Autodesk Inventor part; units mm, degrees
(part 2 of 3)
  line L955 (15.8047, 2.9296) -> (15.8214, 3.0524)
  line L956 (15.8214, 3.0524) -> (15.8318, 3.1132)
  line L957 (15.8318, 3.1132) -> (15.8442, 3.1734)
  line L958 (15.8442, 3.1734) -> (15.5913, 3.315)
  line L959 (15.5913, 3.315) -> (15.2554, 3.4241)
  line L960 (15.2554, 3.4241) -> (14.9676, 3.4583)
  line L961 (14.9676, 3.4583) -> (14.9422, 3.4023)
  line L962 (14.9422, 3.4023) -> (14.915, 3.3469)
  line L963 (14.915, 3.3469) -> (14.8562, 3.2378)
  line L964 (14.8562, 3.2378) -> (14.7929, 3.1303)
  line L965 (14.7929, 3.1303) -> (14.7259, 3.0241)
  line L966 (14.7259, 3.0241) -> (14.5818, 2.8156)
  line L967 (14.5818, 2.8156) -> (14.4261, 2.6115)
  line L968 (14.4261, 2.6115) -> (14.2601, 2.4115)
  line L969 (14.2601, 2.4115) -> (14.0847, 2.2154)
  line L970 (14.0847, 2.2154) -> (13.9004, 2.0233)
  line L971 (13.9004, 2.0233) -> (13.7077, 1.8349)
  line L972 (13.7077, 1.8349) -> (13.507, 1.6503)
  line L973 (13.507, 1.6503) -> (13.3514, 1.5144)
  line L974 (13.3514, 1.5144) -> (12.8549, 1.72)
  line L975 (12.8549, 1.72) -> (12.841, 1.9262)
  line L976 (12.841, 1.9262) -> (12.8296, 2.1986)
  line L977 (12.8296, 2.1986) -> (12.8265, 2.4681)
  line L978 (12.8265, 2.4681) -> (12.8321, 2.7343)
  line L979 (12.8321, 2.7343) -> (12.8466, 2.997)
  line L980 (12.8466, 2.997) -> (12.8707, 3.2557)
  line L981 (12.8707, 3.2557) -> (12.9049, 3.5101)
  line L982 (12.9049, 3.5101) -> (12.9505, 3.7595)
  line L983 (12.9505, 3.7595) -> (12.9781, 3.882)
  line L984 (12.9781, 3.882) -> (13.0095, 4.0027)
  line L985 (13.0095, 4.0027) -> (13.0451, 4.1215)
  line L986 (13.0451, 4.1215) -> (13.0649, 4.1799)
  line L987 (13.0649, 4.1799) -> (13.0865, 4.2374)
  line L988 (13.0865, 4.2374) -> (12.8589, 4.4167)
  line L989 (12.8589, 4.4167) -> (12.5442, 4.5771)
  line L990 (12.5442, 4.5771) -> (12.2654, 4.6558)
  line L991 (12.2654, 4.6558) -> (12.2315, 4.6045)
  line L992 (12.2315, 4.6045) -> (12.1959, 4.5541)
  line L993 (12.1959, 4.5541) -> (12.1208, 4.4555)
  line L994 (12.1208, 4.4555) -> (12.0415, 4.3592)
  line L995 (12.0415, 4.3592) -> (11.9586, 4.2649)
  line L996 (11.9586, 4.2649) -> (11.7837, 4.0814)
  line L997 (11.7837, 4.0814) -> (11.5981, 3.9042)
  line L998 (11.5981, 3.9042) -> (11.4028, 3.7326)
  line L999 (11.4028, 3.7326) -> (11.1989, 3.5664)
  line L1000 (11.1989, 3.5664) -> (10.9868, 3.4055)
  line L1001 (10.9868, 3.4055) -> (10.7669, 3.2496)
  line L1002 (10.7669, 3.2496) -> (10.5398, 3.0987)
  line L1003 (10.5398, 3.0987) -> (10.3649, 2.9888)
  line L1004 (10.3649, 2.9888) -> (9.9067, 3.2695)
  line L1005 (9.9067, 3.2695) -> (9.9252, 3.4753)
  line L1006 (9.9252, 3.4753) -> (9.9566, 3.7462)
  line L1007 (9.9566, 3.7462) -> (9.9957, 4.0128)
  line L1008 (9.9957, 4.0128) -> (10.0428, 4.2749)
  line L1009 (10.0428, 4.2749) -> (10.0983, 4.532)
  line L1010 (10.0983, 4.532) -> (10.1625, 4.7839)
  line L1011 (10.1625, 4.7839) -> (10.2362, 5.0298)
  line L1012 (10.2362, 5.0298) -> (10.3202, 5.2689)
  line L1013 (10.3202, 5.2689) -> (10.3666, 5.3856)
  line L1014 (10.3666, 5.3856) -> (10.4164, 5.5)
  line L1015 (10.4164, 5.5) -> (10.4702, 5.6116)
  line L1016 (10.4702, 5.6116) -> (10.499, 5.6662)
  line L1017 (10.499, 5.6662) -> (10.5293, 5.7197)
  line L1018 (10.5293, 5.7197) -> (10.3326, 5.9324)
  line L1019 (10.3326, 5.9324) -> (10.0468, 6.14)
  line L1020 (10.0468, 6.14) -> (9.7837, 6.2614)
  line L1021 (9.7837, 6.2614) -> (9.7422, 6.216)
  line L1022 (9.7422, 6.216) -> (9.6992, 6.1718)
  line L1023 (9.6992, 6.1718) -> (9.6096, 6.0862)
  line L1024 (9.6096, 6.0862) -> (9.5162, 6.0035)
  line L1025 (9.5162, 6.0035) -> (9.4196, 5.9233)
  line L1026 (9.4196, 5.9233) -> (9.2181, 5.7694)
  line L1027 (9.2181, 5.7694) -> (9.007, 5.6234)
  line L1028 (9.007, 5.6234) -> (8.7874, 5.4845)
  line L1029 (8.7874, 5.4845) -> (8.5599, 5.3523)
  line L1030 (8.5599, 5.3523) -> (8.3252, 5.2265)
  line L1031 (8.3252, 5.2265) -> (8.0837, 5.1069)
  line L1032 (8.0837, 5.1069) -> (7.8358, 4.9934)
  line L1033 (7.8358, 4.9934) -> (7.6459, 4.9122)
  line L1034 (7.6459, 4.9122) -> (7.2372, 5.2611)
  line L1035 (7.2372, 5.2611) -> (7.2877, 5.4615)
  line L1036 (7.2877, 5.4615) -> (7.361, 5.7241)
  line L1037 (7.361, 5.7241) -> (7.4414, 5.9813)
  line L1038 (7.4414, 5.9813) -> (7.5289, 6.2328)
  line L1039 (7.5289, 6.2328) -> (7.6239, 6.4781)
  line L1040 (7.6239, 6.4781) -> (7.7268, 6.7168)
  line L1041 (7.7268, 6.7168) -> (7.838, 6.9482)
  line L1042 (7.838, 6.9482) -> (7.9584, 7.1712)
  line L1043 (7.9584, 7.1712) -> (8.0225, 7.2792)
  line L1044 (8.0225, 7.2792) -> (8.0896, 7.3844)
  line L1045 (8.0896, 7.3844) -> (8.1602, 7.4863)
  line L1046 (8.1602, 7.4863) -> (8.1971, 7.5357)
  line L1047 (8.1971, 7.5357) -> (8.2354, 7.5837)
  line L1048 (8.2354, 7.5837) -> (8.0744, 7.8246)
  line L1049 (8.0744, 7.8246) -> (7.8246, 8.0744)
  line L1050 (7.8246, 8.0744) -> (7.5837, 8.2354)
  line L1051 (7.5837, 8.2354) -> (7.5357, 8.1971)
  line L1052 (7.5357, 8.1971) -> (7.4863, 8.1602)
  line L1053 (7.4863, 8.1602) -> (7.3844, 8.0896)
  line L1054 (7.3844, 8.0896) -> (7.2792, 8.0225)
  line L1055 (7.2792, 8.0225) -> (7.1712, 7.9584)
  line L1056 (7.1712, 7.9584) -> (6.9482, 7.838)
  line L1057 (6.9482, 7.838) -> (6.7168, 7.7268)
  line L1058 (6.7168, 7.7268) -> (6.4781, 7.6239)
  line L1059 (6.4781, 7.6239) -> (6.2328, 7.5289)
  line L1060 (6.2328, 7.5289) -> (5.9813, 7.4414)
  line L1061 (5.9813, 7.4414) -> (5.7241, 7.361)
  line L1062 (5.7241, 7.361) -> (5.4615, 7.2877)
  line L1063 (5.4615, 7.2877) -> (5.2611, 7.2372)
  line L1064 (5.2611, 7.2372) -> (4.9122, 7.6459)
  line L1065 (4.9122, 7.6459) -> (4.9934, 7.8358)
  line L1066 (4.9934, 7.8358) -> (5.1069, 8.0837)
  line L1067 (5.1069, 8.0837) -> (5.2265, 8.3252)
  line L1068 (5.2265, 8.3252) -> (5.3523, 8.5599)
  line L1069 (5.3523, 8.5599) -> (5.4845, 8.7874)
  line L1070 (5.4845, 8.7874) -> (5.6234, 9.007)
  line L1071 (5.6234, 9.007) -> (5.7694, 9.2181)
  line L1072 (5.7694, 9.2181) -> (5.9233, 9.4196)
  line L1073 (5.9233, 9.4196) -> (6.0035, 9.5162)
  line L1074 (6.0035, 9.5162) -> (6.0862, 9.6096)
  line L1075 (6.0862, 9.6096) -> (6.1718, 9.6992)
  line L1076 (6.1718, 9.6992) -> (6.216, 9.7422)
  line L1077 (6.216, 9.7422) -> (6.2614, 9.7837)
  line L1078 (6.2614, 9.7837) -> (6.14, 10.0468)
  line L1079 (6.14, 10.0468) -> (5.9324, 10.3326)
  line L1080 (5.9324, 10.3326) -> (5.7197, 10.5293)
  line L1081 (5.7197, 10.5293) -> (5.6662, 10.499)
  line L1082 (5.6662, 10.499) -> (5.6116, 10.4702)
  line L1083 (5.6116, 10.4702) -> (5.5, 10.4164)
  line L1084 (5.5, 10.4164) -> (5.3856, 10.3666)
  line L1085 (5.3856, 10.3666) -> (5.2689, 10.3202)
  line L1086 (5.2689, 10.3202) -> (5.0298, 10.2362)
  line L1087 (5.0298, 10.2362) -> (4.7839, 10.1625)
  line L1088 (4.7839, 10.1625) -> (4.532, 10.0983)
  line L1089 (4.532, 10.0983) -> (4.2749, 10.0428)
  line L1090 (4.2749, 10.0428) -> (4.0128, 9.9957)
  line L1091 (4.0128, 9.9957) -> (3.7462, 9.9566)
  line L1092 (3.7462, 9.9566) -> (3.4753, 9.9252)
  line L1093 (3.4753, 9.9252) -> (3.2695, 9.9067)
  line L1094 (3.2695, 9.9067) -> (2.9888, 10.3649)
  line L1095 (2.9888, 10.3649) -> (3.0987, 10.5398)
  line L1096 (3.0987, 10.5398) -> (3.2496, 10.7669)
  line L1097 (3.2496, 10.7669) -> (3.4055, 10.9868)
  line L1098 (3.4055, 10.9868) -> (3.5664, 11.1989)
  line L1099 (3.5664, 11.1989) -> (3.7326, 11.4028)
  line L1100 (3.7326, 11.4028) -> (3.9042, 11.5981)
  line L1101 (3.9042, 11.5981) -> (4.0814, 11.7837)
  line L1102 (4.0814, 11.7837) -> (4.2649, 11.9586)
  line L1103 (4.2649, 11.9586) -> (4.3592, 12.0415)
  line L1104 (4.3592, 12.0415) -> (4.4555, 12.1208)
  line L1105 (4.4555, 12.1208) -> (4.5541, 12.1959)
  line L1106 (4.5541, 12.1959) -> (4.6045, 12.2315)
  line L1107 (4.6045, 12.2315) -> (4.6558, 12.2654)
  line L1108 (4.6558, 12.2654) -> (4.5771, 12.5442)
  line L1109 (4.5771, 12.5442) -> (4.4167, 12.8589)
  line L1110 (4.4167, 12.8589) -> (4.2374, 13.0865)
  line L1111 (4.2374, 13.0865) -> (4.1799, 13.0649)
  line L1112 (4.1799, 13.0649) -> (4.1215, 13.0451)
  line L1113 (4.1215, 13.0451) -> (4.0027, 13.0095)
  line L1114 (4.0027, 13.0095) -> (3.882, 12.9781)
  line L1115 (3.882, 12.9781) -> (3.7595, 12.9505)
  line L1116 (3.7595, 12.9505) -> (3.5101, 12.9049)
  line L1117 (3.5101, 12.9049) -> (3.2557, 12.8707)
  line L1118 (3.2557, 12.8707) -> (2.997, 12.8466)
  line L1119 (2.997, 12.8466) -> (2.7343, 12.8321)
  line L1120 (2.7343, 12.8321) -> (2.4681, 12.8265)
  line L1121 (2.4681, 12.8265) -> (2.1986, 12.8296)
  line L1122 (2.1986, 12.8296) -> (1.9262, 12.841)
  line L1123 (1.9262, 12.841) -> (1.72, 12.8549)
  line L1124 (1.72, 12.8549) -> (1.5144, 13.3514)
  line L1125 (1.5144, 13.3514) -> (1.6503, 13.507)
  line L1126 (1.6503, 13.507) -> (1.8349, 13.7077)
  line L1127 (1.8349, 13.7077) -> (2.0233, 13.9004)
  line L1128 (2.0233, 13.9004) -> (2.2154, 14.0847)
  line L1129 (2.2154, 14.0847) -> (2.4115, 14.2601)
  line L1130 (2.4115, 14.2601) -> (2.6115, 14.4261)
  line L1131 (2.6115, 14.4261) -> (2.8156, 14.5818)
  line L1132 (2.8156, 14.5818) -> (3.0241, 14.7259)
  line L1133 (3.0241, 14.7259) -> (3.1303, 14.7929)
  line L1134 (3.1303, 14.7929) -> (3.2378, 14.8562)
  line L1135 (3.2378, 14.8562) -> (3.3469, 14.915)
  line L1136 (3.3469, 14.915) -> (3.4023, 14.9422)
  line L1137 (3.4023, 14.9422) -> (3.4583, 14.9676)
  line L1138 (3.4583, 14.9676) -> (3.4241, 15.2554)
  line L1139 (3.4241, 15.2554) -> (3.315, 15.5913)
  line L1140 (3.315, 15.5913) -> (3.1734, 15.8442)
  line L1141 (3.1734, 15.8442) -> (3.1132, 15.8318)
  line L1142 (3.1132, 15.8318) -> (3.0524, 15.8214)
  line L1143 (3.0524, 15.8214) -> (2.9296, 15.8047)
  line L1144 (2.9296, 15.8047) -> (2.8054, 15.7927)
  line L1145 (2.8054, 15.7927) -> (2.6801, 15.7846)
  line L1146 (2.6801, 15.7846) -> (2.4267, 15.7786)
  line L1147 (2.4267, 15.7786) -> (2.1701, 15.7845)
  line L1148 (2.1701, 15.7845) -> (1.9107, 15.8012)
  line L1149 (1.9107, 15.8012) -> (1.649, 15.828)
  line L1150 (1.649, 15.828) -> (1.3852, 15.8641)
  line L1151 (1.3852, 15.8641) -> (1.1195, 15.9093)
  line L1152 (1.1195, 15.9093) -> (0.8522, 15.9632)
  line L1153 (0.8522, 15.9632) -> (0.6508, 16.0092)
  line L1154 (0.6508, 16.0092) -> (0.5254, 16.5317)
  line L1155 (0.5254, 16.5317) -> (0.684, 16.6641)
  line L1156 (0.684, 16.6641) -> (0.8977, 16.8335)
  line L1157 (0.8977, 16.8335) -> (1.1139, 16.9944)
  line L1158 (1.1139, 16.9944) -> (1.3325, 17.1463)
  line L1159 (1.3325, 17.1463) -> (1.5536, 17.289)
  line L1160 (1.5536, 17.289) -> (1.777, 17.4216)
  line L1161 (1.777, 17.4216) -> (2.003, 17.5434)
  line L1162 (2.003, 17.5434) -> (2.2315, 17.6531)
  line L1163 (2.2315, 17.6531) -> (2.3469, 17.7028)
  line L1164 (2.3469, 17.7028) -> (2.463, 17.7484)
  line L1165 (2.463, 17.7484) -> (2.58, 17.7894)
  line L1166 (2.58, 17.7894) -> (2.6389, 17.8076)
  line L1167 (2.6389, 17.8076) -> (2.6981, 17.824)
  line L1168 (2.6981, 17.824) -> (2.7094, 18.1135)
  line L1169 (2.7094, 18.1135) -> (2.6542, 18.4624)
  line L1170 (2.6542, 18.4624) -> (2.554, 18.7343)
  line L1171 (2.554, 18.7343) -> (2.4925, 18.7315)
  line L1172 (2.4925, 18.7315) -> (2.4309, 18.7307)
  line L1173 (2.4309, 18.7307) -> (2.3069, 18.7335)
  line L1174 (2.3069, 18.7335) -> (2.1824, 18.741)
  line L1175 (2.1824, 18.741) -> (2.0574, 18.7526)
  line L1176 (2.0574, 18.7526) -> (1.8061, 18.7863)
  line L1177 (1.8061, 18.7863) -> (1.5536, 18.8323)
  line L1178 (1.5536, 18.8323) -> (1.3001, 18.8894)
  line L1179 (1.3001, 18.8894) -> (1.0457, 18.9568)
  line L1180 (1.0457, 18.9568) -> (0.7908, 19.0338)
  line L1181 (0.7908, 19.0338) -> (0.5355, 19.1199)
  line L1182 (0.5355, 19.1199) -> (0.2799, 19.215)
  line L1183 (0.2799, 19.215) -> (0.0882, 19.2919)
  line L1184 (0.0882, 19.2919) -> (0.046, 19.8276)
  line L1185 (0.046, 19.8276) -> (0.2234, 19.9336)
  line L1186 (0.2234, 19.9336) -> (0.461, 20.0674)
  line L1187 (0.461, 20.0674) -> (0.6996, 20.1925)
  line L1188 (0.6996, 20.1925) -> (0.9394, 20.3084)
  line L1189 (0.9394, 20.3084) -> (1.18, 20.4147)
  line L1190 (1.18, 20.4147) -> (1.4215, 20.5108)
  line L1191 (1.4215, 20.5108) -> (1.6637, 20.5957)
  line L1192 (1.6637, 20.5957) -> (1.9066, 20.6683)
  line L1193 (1.9066, 20.6683) -> (2.0283, 20.6993)
  line L1194 (2.0283, 20.6993) -> (2.1501, 20.7262)
  line L1195 (2.1501, 20.7262) -> (2.2721, 20.7484)
  line L1196 (2.2721, 20.7484) -> (2.3331, 20.7572)
  line L1197 (2.3331, 20.7572) -> (2.3942, 20.7641)
  line L1198 (2.3942, 20.7641) -> (2.4506, 21.0483)
  line L1199 (2.4506, 21.0483) -> (2.4506, 21.4015)
  circle A0 centre (21.2249, 21.2249) radius 0.5
  line L1200 (0.0671, 22.8901) -> (42.3827, 19.5598) construction
  line L1201 (19.5598, 0.0671) -> (22.8901, 42.3827) construction
  point P0 (21.2249, 21.2249)
derived "Base_part.ipt"
sketch "Sketch10" plane through (0, 0, 0) normal (0, 1, 0) x (-1, 0, 0)
  line L0 (0, 0) -> (0, -14.7228) construction
  line L1 (0, 0) -> (-17.7743, 0) construction
  arc A0 (-17.3183, 4) -> (-17.1952, -4.5) centre (0, 0) ccw
  line L2 (-14.1421, 5) -> (-17.0565, 5)
  line L3 (-14.4568, 4) -> (-17.3183, 4)
  arc A1 (-17.0565, 5) -> (-17.3183, 4) centre (0, 0) ccw
  line L4 (17.1952, 4.5) -> (-17.1952, 4.5) construction
  line L5 (-14.1421, -5) -> (-17.0565, -5)
  line L6 (-14.4568, -4) -> (-17.3183, -4)
  arc A2 (-17.3183, -4) -> (-17.0565, -5) centre (0, 0) ccw
  arc A3 (-5, -17.0565) -> (-4, -17.3183) centre (0, 0) ccw
  line L7 (-5, -14.1421) -> (-5, -17.0565)
  line L8 (-4, -14.4568) -> (-4, -17.3183)
  arc A4 (4, -17.3183) -> (5, -17.0565) centre (0, 0) ccw
  line L9 (4, -14.4568) -> (4, -17.3183)
  line L10 (5, -14.1421) -> (5, -17.0565)
  arc A5 (17.0565, -5) -> (17.3183, -4) centre (0, 0) ccw
  line L11 (14.1421, -5) -> (17.0565, -5)
  line L12 (14.4568, -4) -> (17.3183, -4)
  arc A6 (17.3183, 4) -> (17.0565, 5) centre (0, 0) ccw
  line L13 (14.4568, 4) -> (17.3183, 4)
  line L14 (14.1421, 5) -> (17.0565, 5)
  arc A7 (5, 17.0565) -> (4, 17.3183) centre (0, 0) ccw
  line L15 (5, 14.1421) -> (5, 17.0565)
  line L16 (4, 14.4568) -> (4, 17.3183)
  arc A8 (-4, 17.3183) -> (-5, 17.0565) centre (0, 0) ccw
  line L17 (-4, 14.4568) -> (-4, 17.3183)
  line L18 (-5, 14.1421) -> (-5, 17.0565)
  circle A9 centre (0, 0) radius 17.7743
  circle A10 centre (0, 0) radius 15
  line L19 (-18.7667, -0.5606) -> (-18.8343, -0.2788)
  line L20 (-18.8343, -0.2788) -> (-18.8956, -0.2744)
  line L21 (-18.8956, -0.2744) -> (-18.9569, -0.2679)
  line L22 (-18.9569, -0.2679) -> (-19.0797, -0.2506)
  line L23 (-19.0797, -0.2506) -> (-19.2025, -0.2284)
  line L24 (-19.2025, -0.2284) -> (-19.3252, -0.2022)
  line L25 (-19.3252, -0.2022) -> (-19.5708, -0.1393)
  line L26 (-19.5708, -0.1393) -> (-19.8162, -0.0639)
  line L27 (-19.8162, -0.0639) -> (-20.0612, 0.0226)
  line L28 (-20.0612, 0.0226) -> (-20.3059, 0.1194)
  line L29 (-20.3059, 0.1194) -> (-20.55, 0.2258)
  line L30 (-20.55, 0.2258) -> (-20.7934, 0.3414)
  line L31 (-20.7934, 0.3414) -> (-21.036, 0.4658)
  line L32 (-21.036, 0.4658) -> (-21.2174, 0.5647)
  line L33 (-21.2174, 0.5647) -> (-21.1963, 1.1017)
  line L34 (-21.1963, 1.1017) -> (-21.0077, 1.1861)
  line L35 (-21.0077, 1.1861) -> (-20.7561, 1.2911)
  line L36 (-20.7561, 1.2911) -> (-20.5043, 1.3872)
  line L37 (-20.5043, 1.3872) -> (-20.2526, 1.4742)
  line L38 (-20.2526, 1.4742) -> (-20.0012, 1.5514)
  line L39 (-20.0012, 1.5514) -> (-19.7501, 1.6184)
  line L40 (-19.7501, 1.6184) -> (-19.4995, 1.6743)
  line L41 (-19.4995, 1.6743) -> (-19.2498, 1.7179)
  line L42 (-19.2498, 1.7179) -> (-19.1253, 1.7344)
  line L43 (-19.1253, 1.7344) -> (-19.0012, 1.7468)
  line L44 (-19.0012, 1.7468) -> (-18.8775, 1.7544)
  line L45 (-18.8775, 1.7544) -> (-18.8158, 1.756)
  line L46 (-18.8158, 1.756) -> (-18.7543, 1.7557)
  line L47 (-18.7543, 1.7557) -> (-18.6649, 2.0313)
  line L48 (-18.6649, 2.0313) -> (-18.6234, 2.3821)
  line L49 (-18.6234, 2.3821) -> (-18.646, 2.6709)
  line L50 (-18.646, 2.6709) -> (-18.7059, 2.6849)
  line L51 (-18.7059, 2.6849) -> (-18.7655, 2.7009)
  line L52 (-18.7655, 2.7009) -> (-18.884, 2.7372)
  line L53 (-18.884, 2.7372) -> (-19.0018, 2.7783)
  line L54 (-19.0018, 2.7783) -> (-19.119, 2.8234)
  line L55 (-19.119, 2.8234) -> (-19.3516, 2.924)
  line L56 (-19.3516, 2.924) -> (-19.5822, 3.0368)
  line L57 (-19.5822, 3.0368) -> (-19.8107, 3.1606)
  line L58 (-19.8107, 3.1606) -> (-20.0372, 3.2944)
  line L59 (-20.0372, 3.2944) -> (-20.2616, 3.4377)
  line L60 (-20.2616, 3.4377) -> (-20.484, 3.59)
  line L61 (-20.484, 3.59) -> (-20.7042, 3.7508)
  line L62 (-20.7042, 3.7508) -> (-20.8678, 3.8769)
  line L63 (-20.8678, 3.8769) -> (-20.763, 4.404)
  line L64 (-20.763, 4.404) -> (-20.5635, 4.4578)
  line L65 (-20.5635, 4.4578) -> (-20.2986, 4.5222)
  line L66 (-20.2986, 4.5222) -> (-20.0349, 4.5777)
  line L67 (-20.0349, 4.5777) -> (-19.7727, 4.6242)
  line L68 (-19.7727, 4.6242) -> (-19.5122, 4.6612)
  line L69 (-19.5122, 4.6612) -> (-19.2537, 4.6881)
  line L70 (-19.2537, 4.6881) -> (-18.9975, 4.7041)
  line L71 (-18.9975, 4.7041) -> (-18.7441, 4.708)
  line L72 (-18.7441, 4.708) -> (-18.6186, 4.7049)
  line L73 (-18.6186, 4.7049) -> (-18.494, 4.6977)
  line L74 (-18.494, 4.6977) -> (-18.3706, 4.6859)
  line L75 (-18.3706, 4.6859) -> (-18.3095, 4.6779)
  line L76 (-18.3095, 4.6779) -> (-18.2488, 4.6679)
  line L77 (-18.2488, 4.6679) -> (-18.1173, 4.9261)
  line L78 (-18.1173, 4.9261) -> (-18.0214, 5.2661)
  line L79 (-18.0214, 5.2661) -> (-17.9986, 5.5549)
  line L80 (-17.9986, 5.5549) -> (-18.0556, 5.5781)
  line L81 (-18.0556, 5.5781) -> (-18.1119, 5.6032)
  line L82 (-18.1119, 5.6032) -> (-18.2233, 5.6576)
  line L83 (-18.2233, 5.6576) -> (-18.3332, 5.7166)
  line L84 (-18.3332, 5.7166) -> (-18.4419, 5.7795)
  line L85 (-18.4419, 5.7795) -> (-18.656, 5.9153)
  line L86 (-18.656, 5.9153) -> (-18.866, 6.0628)
  line L87 (-18.866, 6.0628) -> (-19.0724, 6.2208)
  line L88 (-19.0724, 6.2208) -> (-19.2751, 6.3884)
  line L89 (-19.2751, 6.3884) -> (-19.4744, 6.565)
  line L90 (-19.4744, 6.565) -> (-19.6702, 6.7502)
  line L91 (-19.6702, 6.7502) -> (-19.8625, 6.9435)
  line L92 (-19.8625, 6.9435) -> (-20.0044, 7.0936)
  line L93 (-20.0044, 7.0936) -> (-19.8184, 7.5978)
  line L94 (-19.8184, 7.5978) -> (-19.613, 7.6198)
  line L95 (-19.613, 7.6198) -> (-19.3412, 7.6419)
  line L96 (-19.3412, 7.6419) -> (-19.0721, 7.6555)
  line L97 (-19.0721, 7.6555) -> (-18.8059, 7.6604)
  line L98 (-18.8059, 7.6604) -> (-18.5428, 7.6562)
  line L99 (-18.5428, 7.6562) -> (-18.2833, 7.6423)
  line L100 (-18.2833, 7.6423) -> (-18.0278, 7.6181)
  line L101 (-18.0278, 7.6181) -> (-17.7768, 7.5823)
  line L102 (-17.7768, 7.5823) -> (-17.6533, 7.5595)
  line L103 (-17.6533, 7.5595) -> (-17.5314, 7.533)
  line L104 (-17.5314, 7.533) -> (-17.4114, 7.502)
  line L105 (-17.4114, 7.502) -> (-17.3523, 7.4845)
  line L106 (-17.3523, 7.4845) -> (-17.2939, 7.4652)
  line L107 (-17.2939, 7.4652) -> (-17.1237, 7.6996)
  line L108 (-17.1237, 7.6996) -> (-16.9758, 8.0204)
  line L109 (-16.9758, 8.0204) -> (-16.908, 8.3021)
  line L110 (-16.908, 8.3021) -> (-16.9607, 8.334)
  line L111 (-16.9607, 8.334) -> (-17.0124, 8.3676)
  line L112 (-17.0124, 8.3676) -> (-17.1139, 8.4387)
  line L113 (-17.1139, 8.4387) -> (-17.2132, 8.5142)
  line L114 (-17.2132, 8.5142) -> (-17.3107, 8.5933)
  line L115 (-17.3107, 8.5933) -> (-17.5009, 8.7609)
  line L116 (-17.5009, 8.7609) -> (-17.6853, 8.9394)
  line L117 (-17.6853, 8.9394) -> (-17.8644, 9.1278)
  line L118 (-17.8644, 9.1278) -> (-18.0385, 9.325)
  line L119 (-18.0385, 9.325) -> (-18.2076, 9.5307)
  line L120 (-18.2076, 9.5307) -> (-18.3721, 9.7442)
  line L121 (-18.3721, 9.7442) -> (-18.5317, 9.9652)
  line L122 (-18.5317, 9.9652) -> (-18.6485, 10.1357)
  line L123 (-18.6485, 10.1357) -> (-18.3859, 10.6045)
  line L124 (-18.3859, 10.6045) -> (-18.1795, 10.5941)
  line L125 (-18.1795, 10.5941) -> (-17.9077, 10.5734)
  line L126 (-17.9077, 10.5734) -> (-17.6397, 10.5448)
  line L127 (-17.6397, 10.5448) -> (-17.376, 10.508)
  line L128 (-17.376, 10.508) -> (-17.1168, 10.4627)
  line L129 (-17.1168, 10.4627) -> (-16.8627, 10.4084)
  line L130 (-16.8627, 10.4084) -> (-16.6141, 10.3445)
  line L131 (-16.6141, 10.3445) -> (-16.3718, 10.2698)
  line L132 (-16.3718, 10.2698) -> (-16.2534, 10.228)
  line L133 (-16.2534, 10.228) -> (-16.1372, 10.1828)
  line L134 (-16.1372, 10.1828) -> (-16.0235, 10.1334)
  line L135 (-16.0235, 10.1334) -> (-15.9678, 10.1069)
  line L136 (-15.9678, 10.1069) -> (-15.9132, 10.0786)
  line L137 (-15.9132, 10.0786) -> (-15.7084, 10.2836)
  line L138 (-15.7084, 10.2836) -> (-15.5121, 10.5773)
  line L139 (-15.5121, 10.5773) -> (-15.4011, 10.8449)
  line L140 (-15.4011, 10.8449) -> (-15.4481, 10.8846)
  line L141 (-15.4481, 10.8846) -> (-15.494, 10.9259)
  line L142 (-15.494, 10.9259) -> (-15.5831, 11.012)
  line L143 (-15.5831, 11.012) -> (-15.6694, 11.1021)
  line L144 (-15.6694, 11.1021) -> (-15.7533, 11.1955)
  line L145 (-15.7533, 11.1955) -> (-15.915, 11.3908)
  line L146 (-15.915, 11.3908) -> (-16.0692, 11.596)
  line L147 (-16.0692, 11.596) -> (-16.2166, 11.81)
  line L148 (-16.2166, 11.81) -> (-16.3576, 12.0321)
  line L149 (-16.3576, 12.0321) -> (-16.4926, 12.2616)
  line L150 (-16.4926, 12.2616) -> (-16.6215, 12.4982)
  line L151 (-16.6215, 12.4982) -> (-16.7447, 12.7415)
  line L152 (-16.7447, 12.7415) -> (-16.8333, 12.9282)
  line L153 (-16.8333, 12.9282) -> (-16.5006, 13.3502)
  line L154 (-16.5006, 13.3502) -> (-16.2984, 13.3076)
  line L155 (-16.2984, 13.3076) -> (-16.0331, 13.2446)
  line L156 (-16.0331, 13.2446) -> (-15.773, 13.1744)
  line L157 (-15.773, 13.1744) -> (-15.5182, 13.0968)
  line L158 (-15.5182, 13.0968) -> (-15.2694, 13.0115)
  line L159 (-15.2694, 13.0115) -> (-15.0268, 12.9181)
  line L160 (-15.0268, 12.9181) -> (-14.7913, 12.8161)
  line L161 (-14.7913, 12.8161) -> (-14.5637, 12.7045)
  line L162 (-14.5637, 12.7045) -> (-14.4533, 12.6447)
  line L163 (-14.4533, 12.6447) -> (-14.3456, 12.5818)
  line L164 (-14.3456, 12.5818) -> (-14.241, 12.5153)
  line L165 (-14.241, 12.5153) -> (-14.1901, 12.4803)
  line L166 (-14.1901, 12.4803) -> (-14.1406, 12.4439)
  line L167 (-14.1406, 12.4439) -> (-13.9062, 12.6143)
  line L168 (-13.9062, 12.6143) -> (-13.6665, 12.8737)
  line L169 (-13.6665, 12.8737) -> (-13.515, 13.1207)
  line L170 (-13.515, 13.1207) -> (-13.5552, 13.1672)
  line L171 (-13.5552, 13.1672) -> (-13.594, 13.2151)
  line L172 (-13.594, 13.2151) -> (-13.6686, 13.3142)
  line L173 (-13.6686, 13.3142) -> (-13.7397, 13.4166)
  line L174 (-13.7397, 13.4166) -> (-13.808, 13.522)
  line L175 (-13.808, 13.522) -> (-13.9371, 13.7402)
  line L176 (-13.9371, 13.7402) -> (-14.0573, 13.967)
  line L177 (-14.0573, 13.967) -> (-14.1694, 14.2014)
  line L178 (-14.1694, 14.2014) -> (-14.274, 14.4428)
  line L179 (-14.274, 14.4428) -> (-14.3714, 14.6907)
  line L180 (-14.3714, 14.6907) -> (-14.4617, 14.9446)
  line L181 (-14.4617, 14.9446) -> (-14.5453, 15.2041)
  line L182 (-14.5453, 15.2041) -> (-14.6036, 15.4023)
  line L183 (-14.6036, 15.4023) -> (-14.209, 15.7671)
  line L184 (-14.209, 15.7671) -> (-14.016, 15.6934)
  line L185 (-14.016, 15.6934) -> (-13.7638, 15.5897)
  line L186 (-13.7638, 15.5897) -> (-13.5178, 15.4797)
  line L187 (-13.5178, 15.4797) -> (-13.2784, 15.3632)
  line L188 (-13.2784, 15.3632) -> (-13.0459, 15.24)
  line L189 (-13.0459, 15.24) -> (-12.821, 15.1098)
  line L190 (-12.821, 15.1098) -> (-12.6043, 14.9722)
  line L191 (-12.6043, 14.9722) -> (-12.397, 14.8264)
  line L192 (-12.397, 14.8264) -> (-12.2973, 14.75)
  line L193 (-12.2973, 14.75) -> (-12.2007, 14.671)
  line L194 (-12.2007, 14.671) -> (-12.1078, 14.589)
  line L195 (-12.1078, 14.589) -> (-12.0631, 14.5465)
  line L196 (-12.0631, 14.5465) -> (-12.0199, 14.5028)
  line L197 (-12.0199, 14.5028) -> (-11.7617, 14.6344)
  line L198 (-11.7617, 14.6344) -> (-11.4843, 14.8531)
  line L199 (-11.4843, 14.8531) -> (-11.2961, 15.0734)
  line L200 (-11.2961, 15.0734) -> (-11.3285, 15.1256)
  line L201 (-11.3285, 15.1256) -> (-11.3594, 15.179)
  line L202 (-11.3594, 15.179) -> (-11.4175, 15.2885)
  line L203 (-11.4175, 15.2885) -> (-11.4717, 15.4008)
  line L204 (-11.4717, 15.4008) -> (-11.5227, 15.5156)
  line L205 (-11.5227, 15.5156) -> (-11.6161, 15.7512)
  line L206 (-11.6161, 15.7512) -> (-11.6993, 15.9941)
  line L207 (-11.6993, 15.9941) -> (-11.7734, 16.2432)
  line L208 (-11.7734, 16.2432) -> (-11.8389, 16.498)
  line L209 (-11.8389, 16.498) -> (-11.8963, 16.758)
  line L210 (-11.8963, 16.758) -> (-11.9459, 17.0229)
  line L211 (-11.9459, 17.0229) -> (-11.9878, 17.2923)
  line L212 (-11.9878, 17.2923) -> (-12.0144, 17.4972)
  line L213 (-12.0144, 17.4972) -> (-11.5676, 17.7957)
  line L214 (-11.5676, 17.7957) -> (-11.3885, 17.6928)
  line L215 (-11.3885, 17.6928) -> (-11.1556, 17.5509)
  line L216 (-11.1556, 17.5509) -> (-10.9299, 17.4037)
  line L217 (-10.9299, 17.4037) -> (-10.7116, 17.2512)
  line L218 (-10.7116, 17.2512) -> (-10.5013, 17.0932)
  line L219 (-10.5013, 17.0932) -> (-10.2994, 16.9294)
  line L220 (-10.2994, 16.9294) -> (-10.107, 16.7596)
  line L221 (-10.107, 16.7596) -> (-9.925, 16.5831)
  line L222 (-9.925, 16.5831) -> (-9.8385, 16.4921)
  line L223 (-9.8385, 16.4921) -> (-9.7554, 16.399)
  line L224 (-9.7554, 16.399) -> (-9.6765, 16.3034)
  line L225 (-9.6765, 16.3034) -> (-9.639, 16.2545)
  line L226 (-9.639, 16.2545) -> (-9.6031, 16.2046)
  line L227 (-9.6031, 16.2046) -> (-9.3276, 16.2942)
  line L228 (-9.3276, 16.2942) -> (-9.0194, 16.4668)
  line L229 (-9.0194, 16.4668) -> (-8.799, 16.6549)
  line L230 (-8.799, 16.6549) -> (-8.8229, 16.7115)
  line L231 (-8.8229, 16.7115) -> (-8.845, 16.7691)
  line L232 (-8.845, 16.7691) -> (-8.8853, 16.8863)
  line L233 (-8.8853, 16.8863) -> (-8.9213, 17.0058)
  line L234 (-8.9213, 17.0058) -> (-8.9537, 17.1271)
  line L235 (-8.9537, 17.1271) -> (-9.009, 17.3745)
  line L236 (-9.009, 17.3745) -> (-9.0533, 17.6273)
  line L237 (-9.0533, 17.6273) -> (-9.0875, 17.885)
  line L238 (-9.0875, 17.885) -> (-9.1123, 18.1469)
  line L239 (-9.1123, 18.1469) -> (-9.1283, 18.4127)
  line L240 (-9.1283, 18.4127) -> (-9.1358, 18.682)
  line L241 (-9.1358, 18.682) -> (-9.1351, 18.9547)
  line L242 (-9.1351, 18.9547) -> (-9.1293, 19.1612)
  line L243 (-9.1293, 19.1612) -> (-8.6413, 19.3862)
  line L244 (-8.6413, 19.3862) -> (-8.4805, 19.2565)
  line L245 (-8.4805, 19.2565) -> (-8.2727, 19.0799)
  line L246 (-8.2727, 19.0799) -> (-8.0727, 18.8993)
  line L247 (-8.0727, 18.8993) -> (-7.881, 18.7145)
  line L248 (-7.881, 18.7145) -> (-7.698, 18.5255)
  line L249 (-7.698, 18.5255) -> (-7.5243, 18.3322)
  line L250 (-7.5243, 18.3322) -> (-7.3608, 18.1343)
  line L251 (-7.3608, 18.1343) -> (-7.2086, 17.9316)
  line L252 (-7.2086, 17.9316) -> (-7.1374, 17.8282)
  line L253 (-7.1374, 17.8282) -> (-7.07, 17.7232)
  line L254 (-7.07, 17.7232) -> (-7.007, 17.6165)
  line L255 (-7.007, 17.6165) -> (-6.9776, 17.5622)
  line L256 (-6.9776, 17.5622) -> (-6.95, 17.5073)
  line L257 (-6.95, 17.5073) -> (-6.6638, 17.5527)
  line L258 (-6.6638, 17.5527) -> (-6.3324, 17.675)
  line L259 (-6.3324, 17.675) -> (-6.0853, 17.8263)
  line L260 (-6.0853, 17.8263) -> (-6.1, 17.886)
  line L261 (-6.1, 17.886) -> (-6.1128, 17.9463)
  line L262 (-6.1128, 17.9463) -> (-6.1343, 18.0684)
  line L263 (-6.1343, 18.0684) -> (-6.1512, 18.192)
  line L264 (-6.1512, 18.192) -> (-6.1642, 18.3169)
  line L265 (-6.1642, 18.3169) -> (-6.1802, 18.5699)
  line L266 (-6.1802, 18.5699) -> (-6.1843, 18.8265)
  line L267 (-6.1843, 18.8265) -> (-6.1778, 19.0864)
  line L268 (-6.1778, 19.0864) -> (-6.1613, 19.3489)
  line L269 (-6.1613, 19.3489) -> (-6.1355, 19.614)
  line L270 (-6.1355, 19.614) -> (-6.1008, 19.8812)
  line L271 (-6.1008, 19.8812) -> (-6.0575, 20.1504)
  line L272 (-6.0575, 20.1504) -> (-6.0194, 20.3535)
  line L273 (-6.0194, 20.3535) -> (-5.5022, 20.4993)
  line L274 (-5.5022, 20.4993) -> (-5.3637, 20.346)
  line L275 (-5.3637, 20.346) -> (-5.1861, 20.1392)
  line L276 (-5.1861, 20.1392) -> (-5.0169, 19.9295)
  line L277 (-5.0169, 19.9295) -> (-4.8564, 19.717)
  line L278 (-4.8564, 19.717) -> (-4.7052, 19.5017)
  line L279 (-4.7052, 19.5017) -> (-4.5639, 19.2836)
  line L280 (-4.5639, 19.2836) -> (-4.4333, 19.0626)
  line L281 (-4.4333, 19.0626) -> (-4.3147, 18.8385)
  line L282 (-4.3147, 18.8385) -> (-4.2606, 18.7252)
  line L283 (-4.2606, 18.7252) -> (-4.2104, 18.611)
  line L284 (-4.2104, 18.611) -> (-4.1649, 18.4957)
  line L285 (-4.1649, 18.4957) -> (-4.1443, 18.4376)
  line L286 (-4.1443, 18.4376) -> (-4.1257, 18.379)
  line L287 (-4.1257, 18.379) -> (-3.8359, 18.3791)
  line L288 (-3.8359, 18.3791) -> (-3.4895, 18.448)
  line L289 (-3.4895, 18.448) -> (-3.2217, 18.5588)
  line L290 (-3.2217, 18.5588) -> (-3.2269, 18.62)
  line L291 (-3.2269, 18.62) -> (-3.2301, 18.6816)
  line L292 (-3.2301, 18.6816) -> (-3.2322, 18.8056)
  line L293 (-3.2322, 18.8056) -> (-3.2296, 18.9303)
  line L294 (-3.2296, 18.9303) -> (-3.2229, 19.0557)
  line L295 (-3.2229, 19.0557) -> (-3.1991, 19.3081)
  line L296 (-3.1991, 19.3081) -> (-3.163, 19.5622)
  line L297 (-3.163, 19.5622) -> (-3.1159, 19.8178)
  line L298 (-3.1159, 19.8178) -> (-3.0586, 20.0746)
  line L299 (-3.0586, 20.0746) -> (-2.9917, 20.3323)
  line L300 (-2.9917, 20.3323) -> (-2.9156, 20.5908)
  line L301 (-2.9156, 20.5908) -> (-2.8307, 20.8499)
  line L302 (-2.8307, 20.8499) -> (-2.7614, 21.0445)
  line L303 (-2.7614, 21.0445) -> (-2.2277, 21.1077)
  line L304 (-2.2277, 21.1077) -> (-2.1148, 20.9346)
  line L305 (-2.1148, 20.9346) -> (-1.9718, 20.7025)
  line L306 (-1.9718, 20.7025) -> (-1.8374, 20.4689)
  line L307 (-1.8374, 20.4689) -> (-1.7122, 20.2339)
  line L308 (-1.7122, 20.2339) -> (-1.5965, 19.9976)
  line L309 (-1.5965, 19.9976) -> (-1.4911, 19.7601)
  line L310 (-1.4911, 19.7601) -> (-1.3967, 19.5214)
  line L311 (-1.3967, 19.5214) -> (-1.3146, 19.2815)
  line L312 (-1.3146, 19.2815) -> (-1.2789, 19.1612)
  line L313 (-1.2789, 19.1612) -> (-1.2472, 19.0405)
  line L314 (-1.2472, 19.0405) -> (-1.2203, 18.9195)
  line L315 (-1.2203, 18.9195) -> (-1.209, 18.8589)
  line L316 (-1.209, 18.8589) -> (-1.1998, 18.7981)
  line L317 (-1.1998, 18.7981) -> (-0.9135, 18.7529)
  line L318 (-0.9135, 18.7529) -> (-0.5606, 18.7667)
  line L319 (-0.5606, 18.7667) -> (-0.2788, 18.8343)
  line L320 (-0.2788, 18.8343) -> (-0.2744, 18.8956)
  line L321 (-0.2744, 18.8956) -> (-0.2679, 18.9569)
  line L322 (-0.2679, 18.9569) -> (-0.2506, 19.0797)
  line L323 (-0.2506, 19.0797) -> (-0.2284, 19.2025)
  line L324 (-0.2284, 19.2025) -> (-0.2022, 19.3252)
  line L325 (-0.2022, 19.3252) -> (-0.1393, 19.5708)
  line L326 (-0.1393, 19.5708) -> (-0.0639, 19.8162)
  line L327 (-0.0639, 19.8162) -> (0.0226, 20.0612)
  line L328 (0.0226, 20.0612) -> (0.1194, 20.3059)
  line L329 (0.1194, 20.3059) -> (0.2258, 20.55)
  line L330 (0.2258, 20.55) -> (0.3414, 20.7934)
  line L331 (0.3414, 20.7934) -> (0.4658, 21.036)
  line L332 (0.4658, 21.036) -> (0.5647, 21.2174)
  line L333 (0.5647, 21.2174) -> (1.1017, 21.1963)
  line L334 (1.1017, 21.1963) -> (1.1861, 21.0077)
  line L335 (1.1861, 21.0077) -> (1.2911, 20.7561)
  line L336 (1.2911, 20.7561) -> (1.3872, 20.5043)
  line L337 (1.3872, 20.5043) -> (1.4742, 20.2526)
  line L338 (1.4742, 20.2526) -> (1.5514, 20.0012)
  line L339 (1.5514, 20.0012) -> (1.6184, 19.7501)
  line L340 (1.6184, 19.7501) -> (1.6743, 19.4995)
  line L341 (1.6743, 19.4995) -> (1.7179, 19.2498)
  line L342 (1.7179, 19.2498) -> (1.7344, 19.1253)
  line L343 (1.7344, 19.1253) -> (1.7468, 19.0012)
  line L344 (1.7468, 19.0012) -> (1.7544, 18.8775)
  line L345 (1.7544, 18.8775) -> (1.756, 18.8158)
  line L346 (1.756, 18.8158) -> (1.7557, 18.7543)
  line L347 (1.7557, 18.7543) -> (2.0313, 18.6649)
  line L348 (2.0313, 18.6649) -> (2.3821, 18.6234)
  line L349 (2.3821, 18.6234) -> (2.6709, 18.646)
  line L350 (2.6709, 18.646) -> (2.6849, 18.7059)
  line L351 (2.6849, 18.7059) -> (2.7009, 18.7655)
  line L352 (2.7009, 18.7655) -> (2.7372, 18.884)
  line L353 (2.7372, 18.884) -> (2.7783, 19.0018)
  line L354 (2.7783, 19.0018) -> (2.8234, 19.119)
  line L355 (2.8234, 19.119) -> (2.924, 19.3516)
  line L356 (2.924, 19.3516) -> (3.0368, 19.5822)
  line L357 (3.0368, 19.5822) -> (3.1606, 19.8107)
  line L358 (3.1606, 19.8107) -> (3.2944, 20.0372)
  line L359 (3.2944, 20.0372) -> (3.4377, 20.2616)
  line L360 (3.4377, 20.2616) -> (3.59, 20.484)
  line L361 (3.59, 20.484) -> (3.7508, 20.7042)
  line L362 (3.7508, 20.7042) -> (3.8769, 20.8678)
  line L363 (3.8769, 20.8678) -> (4.404, 20.763)
  line L364 (4.404, 20.763) -> (4.4578, 20.5635)
  line L365 (4.4578, 20.5635) -> (4.5222, 20.2986)
  line L366 (4.5222, 20.2986) -> (4.5777, 20.0349)
  line L367 (4.5777, 20.0349) -> (4.6242, 19.7727)
  line L368 (4.6242, 19.7727) -> (4.6612, 19.5122)
  line L369 (4.6612, 19.5122) -> (4.6881, 19.2537)
  line L370 (4.6881, 19.2537) -> (4.7041, 18.9975)
  line L371 (4.7041, 18.9975) -> (4.708, 18.7441)
  line L372 (4.708, 18.7441) -> (4.7049, 18.6186)
  line L373 (4.7049, 18.6186) -> (4.6977, 18.494)
  line L374 (4.6977, 18.494) -> (4.6859, 18.3706)
  line L375 (4.6859, 18.3706) -> (4.6779, 18.3095)
  line L376 (4.6779, 18.3095) -> (4.6679, 18.2488)
  line L377 (4.6679, 18.2488) -> (4.9261, 18.1173)
  line L378 (4.9261, 18.1173) -> (5.2661, 18.0215)
  line L379 (5.2661, 18.0215) -> (5.5549, 17.9986)
  line L380 (5.5549, 17.9986) -> (5.5781, 18.0556)
  line L381 (5.5781, 18.0556) -> (5.6032, 18.1119)
  line L382 (5.6032, 18.1119) -> (5.6576, 18.2233)
  line L383 (5.6576, 18.2233) -> (5.7166, 18.3332)
  line L384 (5.7166, 18.3332) -> (5.7795, 18.4419)
  line L385 (5.7795, 18.4419) -> (5.9153, 18.656)
  line L386 (5.9153, 18.656) -> (6.0628, 18.866)
  line L387 (6.0628, 18.866) -> (6.2208, 19.0724)
  line L388 (6.2208, 19.0724) -> (6.3884, 19.2751)
  line L389 (6.3884, 19.2751) -> (6.565, 19.4744)
  line L390 (6.565, 19.4744) -> (6.7502, 19.6702)
  line L391 (6.7502, 19.6702) -> (6.9435, 19.8625)
  line L392 (6.9435, 19.8625) -> (7.0936, 20.0044)
  line L393 (7.0936, 20.0044) -> (7.5978, 19.8184)
  line L394 (7.5978, 19.8184) -> (7.6198, 19.613)
  line L395 (7.6198, 19.613) -> (7.6419, 19.3412)
  line L396 (7.6419, 19.3412) -> (7.6555, 19.0721)
  line L397 (7.6555, 19.0721) -> (7.6604, 18.8059)
  line L398 (7.6604, 18.8059) -> (7.6562, 18.5428)
  line L399 (7.6562, 18.5428) -> (7.6423, 18.2833)
  line L400 (7.6423, 18.2833) -> (7.6181, 18.0278)
  line L401 (7.6181, 18.0278) -> (7.5823, 17.7768)
  line L402 (7.5823, 17.7768) -> (7.5595, 17.6533)
  line L403 (7.5595, 17.6533) -> (7.533, 17.5314)
  line L404 (7.533, 17.5314) -> (7.502, 17.4114)
  line L405 (7.502, 17.4114) -> (7.4845, 17.3523)
  line L406 (7.4845, 17.3523) -> (7.4652, 17.2939)
  line L407 (7.4652, 17.2939) -> (7.6996, 17.1237)
  line L408 (7.6996, 17.1237) -> (8.0204, 16.9758)
  line L409 (8.0204, 16.9758) -> (8.3021, 16.9081)
  line L410 (8.3021, 16.9081) -> (8.334, 16.9607)
  line L411 (8.334, 16.9607) -> (8.3675, 17.0124)
  line L412 (8.3675, 17.0124) -> (8.4387, 17.1139)
  line L413 (8.4387, 17.1139) -> (8.5142, 17.2132)
  line L414 (8.5142, 17.2132) -> (8.5933, 17.3107)
  line L415 (8.5933, 17.3107) -> (8.7609, 17.5009)
  line L416 (8.7609, 17.5009) -> (8.9394, 17.6853)
  line L417 (8.9394, 17.6853) -> (9.1278, 17.8644)
  line L418 (9.1278, 17.8644) -> (9.325, 18.0385)
  line L419 (9.325, 18.0385) -> (9.5307, 18.2076)
  line L420 (9.5307, 18.2076) -> (9.7442, 18.3721)
  line L421 (9.7442, 18.3721) -> (9.9652, 18.5318)
  line L422 (9.9652, 18.5318) -> (10.1357, 18.6484)
  line L423 (10.1357, 18.6484) -> (10.6045, 18.3859)
  line L424 (10.6045, 18.3859) -> (10.5941, 18.1795)
  line L425 (10.5941, 18.1795) -> (10.5734, 17.9077)
  line L426 (10.5734, 17.9077) -> (10.5448, 17.6397)
  line L427 (10.5448, 17.6397) -> (10.508, 17.376)
  line L428 (10.508, 17.376) -> (10.4627, 17.1168)
  line L429 (10.4627, 17.1168) -> (10.4084, 16.8627)
  line L430 (10.4084, 16.8627) -> (10.3445, 16.6141)
  line L431 (10.3445, 16.6141) -> (10.2698, 16.3718)
  line L432 (10.2698, 16.3718) -> (10.228, 16.2534)
  line L433 (10.228, 16.2534) -> (10.1828, 16.1372)
  line L434 (10.1828, 16.1372) -> (10.1334, 16.0235)
  line L435 (10.1334, 16.0235) -> (10.1069, 15.9678)
  line L436 (10.1069, 15.9678) -> (10.0786, 15.9132)
  line L437 (10.0786, 15.9132) -> (10.2836, 15.7083)
  line L438 (10.2836, 15.7083) -> (10.5773, 15.5121)
  line L439 (10.5773, 15.5121) -> (10.8449, 15.4011)
  line L440 (10.8449, 15.4011) -> (10.8846, 15.4481)
  line L441 (10.8846, 15.4481) -> (10.9259, 15.494)
  line L442 (10.9259, 15.494) -> (11.012, 15.5831)
  line L443 (11.012, 15.5831) -> (11.1021, 15.6694)
  line L444 (11.1021, 15.6694) -> (11.1955, 15.7533)
  line L445 (11.1955, 15.7533) -> (11.3908, 15.915)
  line L446 (11.3908, 15.915) -> (11.596, 16.0692)
  line L447 (11.596, 16.0692) -> (11.81, 16.2166)
  line L448 (11.81, 16.2166) -> (12.0321, 16.3576)
  line L449 (12.0321, 16.3576) -> (12.2616, 16.4926)
  line L450 (12.2616, 16.4926) -> (12.4982, 16.6215)
  line L451 (12.4982, 16.6215) -> (12.7415, 16.7447)
  line L452 (12.7415, 16.7447) -> (12.9282, 16.8333)
  line L453 (12.9282, 16.8333) -> (13.3502, 16.5006)
  line L454 (13.3502, 16.5006) -> (13.3076, 16.2984)
  line L455 (13.3076, 16.2984) -> (13.2446, 16.0331)
  line L456 (13.2446, 16.0331) -> (13.1744, 15.773)
  line L457 (13.1744, 15.773) -> (13.0968, 15.5182)
  line L458 (13.0968, 15.5182) -> (13.0115, 15.2694)
  line L459 (13.0115, 15.2694) -> (12.9181, 15.0268)
  line L460 (12.9181, 15.0268) -> (12.8161, 14.7913)
  line L461 (12.8161, 14.7913) -> (12.7045, 14.5637)
  line L462 (12.7045, 14.5637) -> (12.6447, 14.4533)
  line L463 (12.6447, 14.4533) -> (12.5818, 14.3456)
  line L464 (12.5818, 14.3456) -> (12.5153, 14.241)
  line L465 (12.5153, 14.241) -> (12.4803, 14.1901)
  line L466 (12.4803, 14.1901) -> (12.4439, 14.1406)
  line L467 (12.4439, 14.1406) -> (12.6143, 13.9062)
  line L468 (12.6143, 13.9062) -> (12.8737, 13.6665)
  line L469 (12.8737, 13.6665) -> (13.1207, 13.515)
  line L470 (13.1207, 13.515) -> (13.1672, 13.5552)
  line L471 (13.1672, 13.5552) -> (13.2151, 13.594)
  line L472 (13.2151, 13.594) -> (13.3142, 13.6686)
  line L473 (13.3142, 13.6686) -> (13.4166, 13.7397)
  line L474 (13.4166, 13.7397) -> (13.522, 13.808)
  line L475 (13.522, 13.808) -> (13.7402, 13.9371)
  line L476 (13.7402, 13.9371) -> (13.967, 14.0573)
  line L477 (13.967, 14.0573) -> (14.2014, 14.1694)
  line L478 (14.2014, 14.1694) -> (14.4428, 14.274)
  line L479 (14.4428, 14.274) -> (14.6907, 14.3714)
  line L480 (14.6907, 14.3714) -> (14.9445, 14.4617)
  line L481 (14.9445, 14.4617) -> (15.2041, 14.5453)
  line L482 (15.2041, 14.5453) -> (15.4023, 14.6036)
  line L483 (15.4023, 14.6036) -> (15.7671, 14.209)
  line L484 (15.7671, 14.209) -> (15.6934, 14.016)
  line L485 (15.6934, 14.016) -> (15.5897, 13.7638)
  line L486 (15.5897, 13.7638) -> (15.4797, 13.5178)
  line L487 (15.4797, 13.5178) -> (15.3632, 13.2784)
  line L488 (15.3632, 13.2784) -> (15.24, 13.0459)
  line L489 (15.24, 13.0459) -> (15.1098, 12.821)
  line L490 (15.1098, 12.821) -> (14.9722, 12.6043)
  line L491 (14.9722, 12.6043) -> (14.8264, 12.397)
  line L492 (14.8264, 12.397) -> (14.75, 12.2973)
  line L493 (14.75, 12.2973) -> (14.671, 12.2007)
  line L494 (14.671, 12.2007) -> (14.589, 12.1078)
  line L495 (14.589, 12.1078) -> (14.5465, 12.0631)
  line L496 (14.5465, 12.0631) -> (14.5028, 12.0199)
  line L497 (14.5028, 12.0199) -> (14.6344, 11.7617)
  line L498 (14.6344, 11.7617) -> (14.8531, 11.4843)
  line L499 (14.8531, 11.4843) -> (15.0734, 11.2961)
  line L500 (15.0734, 11.2961) -> (15.1256, 11.3285)
  line L501 (15.1256, 11.3285) -> (15.179, 11.3594)
  line L502 (15.179, 11.3594) -> (15.2885, 11.4175)
  line L503 (15.2885, 11.4175) -> (15.4008, 11.4717)
  line L504 (15.4008, 11.4717) -> (15.5156, 11.5227)
  line L505 (15.5156, 11.5227) -> (15.7512, 11.6161)
  line L506 (15.7512, 11.6161) -> (15.9941, 11.6993)
  line L507 (15.9941, 11.6993) -> (16.2432, 11.7734)
  line L508 (16.2432, 11.7734) -> (16.498, 11.8389)
  line L509 (16.498, 11.8389) -> (16.758, 11.8963)
  line L510 (16.758, 11.8963) -> (17.0229, 11.9459)
  line L511 (17.0229, 11.9459) -> (17.2923, 11.9878)
  line L512 (17.2923, 11.9878) -> (17.4972, 12.0144)
  line L513 (17.4972, 12.0144) -> (17.7957, 11.5676)
  line L514 (17.7957, 11.5676) -> (17.6928, 11.3885)
  line L515 (17.6928, 11.3885) -> (17.5509, 11.1556)
  line L516 (17.5509, 11.1556) -> (17.4037, 10.9299)
  line L517 (17.4037, 10.9299) -> (17.2512, 10.7116)
  line L518 (17.2512, 10.7116) -> (17.0932, 10.5012)
  line L519 (17.0932, 10.5012) -> (16.9294, 10.2995)
  line L520 (16.9294, 10.2995) -> (16.7596, 10.107)
  line L521 (16.7596, 10.107) -> (16.5831, 9.925)
  line L522 (16.5831, 9.925) -> (16.4921, 9.8385)
  line L523 (16.4921, 9.8385) -> (16.399, 9.7554)
  line L524 (16.399, 9.7554) -> (16.3034, 9.6765)
  line L525 (16.3034, 9.6765) -> (16.2545, 9.639)
  line L526 (16.2545, 9.639) -> (16.2045, 9.6031)
  line L527 (16.2045, 9.6031) -> (16.2942, 9.3276)
  line L528 (16.2942, 9.3276) -> (16.4668, 9.0194)
  line L529 (16.4668, 9.0194) -> (16.6549, 8.799)
  line L530 (16.6549, 8.799) -> (16.7115, 8.8229)
  line L531 (16.7115, 8.8229) -> (16.7691, 8.845)
  line L532 (16.7691, 8.845) -> (16.8863, 8.8853)
  line L533 (16.8863, 8.8853) -> (17.0058, 8.9213)
  line L534 (17.0058, 8.9213) -> (17.1271, 8.9537)
  line L535 (17.1271, 8.9537) -> (17.3745, 9.009)
  line L536 (17.3745, 9.009) -> (17.6273, 9.0533)
  line L537 (17.6273, 9.0533) -> (17.885, 9.0875)
  line L538 (17.885, 9.0875) -> (18.1469, 9.1123)
  line L539 (18.1469, 9.1123) -> (18.4127, 9.1283)
  line L540 (18.4127, 9.1283) -> (18.682, 9.1358)
  line L541 (18.682, 9.1358) -> (18.9547, 9.1351)
  line L542 (18.9547, 9.1351) -> (19.1612, 9.1293)
  line L543 (19.1612, 9.1293) -> (19.3862, 8.6413)
  line L544 (19.3862, 8.6413) -> (19.2565, 8.4805)
  line L545 (19.2565, 8.4805) -> (19.0799, 8.2727)
  line L546 (19.0799, 8.2727) -> (18.8993, 8.0727)
  line L547 (18.8993, 8.0727) -> (18.7145, 7.881)
  line L548 (18.7145, 7.881) -> (18.5255, 7.698)
  line L549 (18.5255, 7.698) -> (18.3322, 7.5243)
  line L550 (18.3322, 7.5243) -> (18.1343, 7.3608)
  line L551 (18.1343, 7.3608) -> (17.9316, 7.2086)
  line L552 (17.9316, 7.2086) -> (17.8282, 7.1374)
  line L553 (17.8282, 7.1374) -> (17.7232, 7.07)
  line L554 (17.7232, 7.07) -> (17.6165, 7.007)
  line L555 (17.6165, 7.007) -> (17.5622, 6.9776)
  line L556 (17.5622, 6.9776) -> (17.5073, 6.95)
  line L557 (17.5073, 6.95) -> (17.5527, 6.6638)
  line L558 (17.5527, 6.6638) -> (17.675, 6.3324)
  line L559 (17.675, 6.3324) -> (17.8263, 6.0853)
  line L560 (17.8263, 6.0853) -> (17.886, 6.1)
  line L561 (17.886, 6.1) -> (17.9463, 6.1128)
  line L562 (17.9463, 6.1128) -> (18.0684, 6.1343)
  line L563 (18.0684, 6.1343) -> (18.192, 6.1512)
  line L564 (18.192, 6.1512) -> (18.3169, 6.1642)
  line L565 (18.3169, 6.1642) -> (18.5699, 6.1802)
  line L566 (18.5699, 6.1802) -> (18.8265, 6.1843)
  line L567 (18.8265, 6.1843) -> (19.0863, 6.1778)
  line L568 (19.0863, 6.1778) -> (19.3489, 6.1613)
  line L569 (19.3489, 6.1613) -> (19.614, 6.1355)
  line L570 (19.614, 6.1355) -> (19.8812, 6.1008)
  line L571 (19.8812, 6.1008) -> (20.1504, 6.0575)
  line L572 (20.1504, 6.0575) -> (20.3535, 6.0194)
  line L573 (20.3535, 6.0194) -> (20.4993, 5.5022)
  line L574 (20.4993, 5.5022) -> (20.346, 5.3637)
  line L575 (20.346, 5.3637) -> (20.1392, 5.1861)
  line L576 (20.1392, 5.1861) -> (19.9295, 5.0169)
  line L577 (19.9295, 5.0169) -> (19.717, 4.8564)
  line L578 (19.717, 4.8564) -> (19.5017, 4.7052)
  line L579 (19.5017, 4.7052) -> (19.2836, 4.5639)
  line L580 (19.2836, 4.5639) -> (19.0626, 4.4333)
  line L581 (19.0626, 4.4333) -> (18.8385, 4.3147)
  line L582 (18.8385, 4.3147) -> (18.7252, 4.2606)
  line L583 (18.7252, 4.2606) -> (18.611, 4.2104)
  line L584 (18.611, 4.2104) -> (18.4957, 4.1649)
  line L585 (18.4957, 4.1649) -> (18.4376, 4.1443)
  line L586 (18.4376, 4.1443) -> (18.379, 4.1257)
  line L587 (18.379, 4.1257) -> (18.3791, 3.8359)
  line L588 (18.3791, 3.8359) -> (18.448, 3.4895)
  line L589 (18.448, 3.4895) -> (18.5588, 3.2217)
  line L590 (18.5588, 3.2217) -> (18.62, 3.2269)
  line L591 (18.62, 3.2269) -> (18.6816, 3.2301)
  line L592 (18.6816, 3.2301) -> (18.8056, 3.2322)
  line L593 (18.8056, 3.2322) -> (18.9303, 3.2296)
  line L594 (18.9303, 3.2296) -> (19.0557, 3.2229)
  line L595 (19.0557, 3.2229) -> (19.3081, 3.1991)
  line L596 (19.3081, 3.1991) -> (19.5622, 3.163)
  line L597 (19.5622, 3.163) -> (19.8178, 3.1159)
  line L598 (19.8178, 3.1159) -> (20.0745, 3.0586)
  line L599 (20.0745, 3.0586) -> (20.3323, 2.9917)
  line L600 (20.3323, 2.9917) -> (20.5908, 2.9156)
  line L601 (20.5908, 2.9156) -> (20.8499, 2.8307)
  line L602 (20.8499, 2.8307) -> (21.0445, 2.7613)
  line L603 (21.0445, 2.7613) -> (21.1077, 2.2277)
  line L604 (21.1077, 2.2277) -> (20.9346, 2.1148)
  line L605 (20.9346, 2.1148) -> (20.7025, 1.9718)
  line L606 (20.7025, 1.9718) -> (20.4689, 1.8374)
  line L607 (20.4689, 1.8374) -> (20.2339, 1.7122)
  line L608 (20.2339, 1.7122) -> (19.9976, 1.5965)
  line L609 (19.9976, 1.5965) -> (19.7601, 1.4911)
  line L610 (19.7601, 1.4911) -> (19.5214, 1.3967)
  line L611 (19.5214, 1.3967) -> (19.2815, 1.3146)
  line L612 (19.2815, 1.3146) -> (19.1612, 1.2789)
  line L613 (19.1612, 1.2789) -> (19.0405, 1.2472)
  line L614 (19.0405, 1.2472) -> (18.9195, 1.2203)
  line L615 (18.9195, 1.2203) -> (18.8589, 1.209)
  line L616 (18.8589, 1.209) -> (18.7981, 1.1998)
  line L617 (18.7981, 1.1998) -> (18.7529, 0.9135)
  line L618 (18.7529, 0.9135) -> (18.7667, 0.5606)
  line L619 (18.7667, 0.5606) -> (18.8343, 0.2788)
  line L620 (18.8343, 0.2788) -> (18.8956, 0.2744)
  line L621 (18.8956, 0.2744) -> (18.9569, 0.2679)
  line L622 (18.9569, 0.2679) -> (19.0797, 0.2506)
  line L623 (19.0797, 0.2506) -> (19.2024, 0.2285)
  line L624 (19.2024, 0.2285) -> (19.3252, 0.2022)
  line L625 (19.3252, 0.2022) -> (19.5708, 0.1393)
  line L626 (19.5708, 0.1393) -> (19.8162, 0.0639)
  line L627 (19.8162, 0.0639) -> (20.0612, -0.0226)
  line L628 (20.0612, -0.0226) -> (20.3059, -0.1194)
  line L629 (20.3059, -0.1194) -> (20.55, -0.2258)
  line L630 (20.55, -0.2258) -> (20.7934, -0.3414)
  line L631 (20.7934, -0.3414) -> (21.036, -0.4658)
  line L632 (21.036, -0.4658) -> (21.2174, -0.5647)
  line L633 (21.2174, -0.5647) -> (21.1963, -1.1017)
  line L634 (21.1963, -1.1017) -> (21.0077, -1.1861)
  line L635 (21.0077, -1.1861) -> (20.7561, -1.2911)
  line L636 (20.7561, -1.2911) -> (20.5043, -1.3872)
  line L637 (20.5043, -1.3872) -> (20.2526, -1.4742)
  line L638 (20.2526, -1.4742) -> (20.0012, -1.5514)
  line L639 (20.0012, -1.5514) -> (19.7501, -1.6184)
  line L640 (19.7501, -1.6184) -> (19.4995, -1.6743)
  line L641 (19.4995, -1.6743) -> (19.2498, -1.7179)
  line L642 (19.2498, -1.7179) -> (19.1253, -1.7343)
  line L643 (19.1253, -1.7343) -> (19.0012, -1.7468)
  line L644 (19.0012, -1.7468) -> (18.8775, -1.7544)
  line L645 (18.8775, -1.7544) -> (18.8158, -1.756)
  line L646 (18.8158, -1.756) -> (18.7543, -1.7557)
  line L647 (18.7543, -1.7557) -> (18.6649, -2.0313)
  line L648 (18.6649, -2.0313) -> (18.6234, -2.3821)
  line L649 (18.6234, -2.3821) -> (18.646, -2.6709)
  line L650 (18.646, -2.6709) -> (18.7059, -2.6849)
  line L651 (18.7059, -2.6849) -> (18.7655, -2.7009)
  line L652 (18.7655, -2.7009) -> (18.884, -2.7372)
  line L653 (18.884, -2.7372) -> (19.0018, -2.7783)
  line L654 (19.0018, -2.7783) -> (19.119, -2.8234)
  line L655 (19.119, -2.8234) -> (19.3516, -2.924)
  line L656 (19.3516, -2.924) -> (19.5822, -3.0368)
  line L657 (19.5822, -3.0368) -> (19.8107, -3.1606)
  line L658 (19.8107, -3.1606) -> (20.0372, -3.2944)
  line L659 (20.0372, -3.2944) -> (20.2616, -3.4377)
  line L660 (20.2616, -3.4377) -> (20.484, -3.59)
  line L661 (20.484, -3.59) -> (20.7042, -3.7508)
  line L662 (20.7042, -3.7508) -> (20.8678, -3.8769)
  line L663 (20.8678, -3.8769) -> (20.763, -4.404)
  line L664 (20.763, -4.404) -> (20.5635, -4.4578)
  line L665 (20.5635, -4.4578) -> (20.2986, -4.5222)
  line L666 (20.2986, -4.5222) -> (20.0349, -4.5777)
  line L667 (20.0349, -4.5777) -> (19.7727, -4.6242)
  line L668 (19.7727, -4.6242) -> (19.5122, -4.6612)
  line L669 (19.5122, -4.6612) -> (19.2537, -4.6881)
  line L670 (19.2537, -4.6881) -> (18.9975, -4.7041)
  line L671 (18.9975, -4.7041) -> (18.7441, -4.708)
  line L672 (18.7441, -4.708) -> (18.6186, -4.7049)
  line L673 (18.6186, -4.7049) -> (18.494, -4.6977)
  line L674 (18.494, -4.6977) -> (18.3706, -4.6859)
  line L675 (18.3706, -4.6859) -> (18.3095, -4.6779)
  line L676 (18.3095, -4.6779) -> (18.2488, -4.6679)
  line L677 (18.2488, -4.6679) -> (18.1173, -4.9261)
  line L678 (18.1173, -4.9261) -> (18.0215, -5.2661)
  line L679 (18.0215, -5.2661) -> (17.9986, -5.5549)
  line L680 (17.9986, -5.5549) -> (18.0556, -5.5781)
  line L681 (18.0556, -5.5781) -> (18.1119, -5.6032)
  line L682 (18.1119, -5.6032) -> (18.2233, -5.6576)
  line L683 (18.2233, -5.6576) -> (18.3332, -5.7166)
  line L684 (18.3332, -5.7166) -> (18.4419, -5.7795)
  line L685 (18.4419, -5.7795) -> (18.656, -5.9153)
  line L686 (18.656, -5.9153) -> (18.866, -6.0628)
  line L687 (18.866, -6.0628) -> (19.0724, -6.2208)
  line L688 (19.0724, -6.2208) -> (19.2751, -6.3884)
  line L689 (19.2751, -6.3884) -> (19.4744, -6.565)
  line L690 (19.4744, -6.565) -> (19.6702, -6.7502)
  line L691 (19.6702, -6.7502) -> (19.8625, -6.9435)
  line L692 (19.8625, -6.9435) -> (20.0044, -7.0936)
  line L693 (20.0044, -7.0936) -> (19.8184, -7.5978)
  line L694 (19.8184, -7.5978) -> (19.613, -7.6198)
  line L695 (19.613, -7.6198) -> (19.3412, -7.6419)
  line L696 (19.3412, -7.6419) -> (19.0721, -7.6555)
  line L697 (19.0721, -7.6555) -> (18.8059, -7.6604)
  line L698 (18.8059, -7.6604) -> (18.5428, -7.6562)
  line L699 (18.5428, -7.6562) -> (18.2833, -7.6423)
  line L700 (18.2833, -7.6423) -> (18.0278, -7.6181)
  line L701 (18.0278, -7.6181) -> (17.7768, -7.5823)
  line L702 (17.7768, -7.5823) -> (17.6533, -7.5595)
  line L703 (17.6533, -7.5595) -> (17.5314, -7.533)
  line L704 (17.5314, -7.533) -> (17.4114, -7.502)